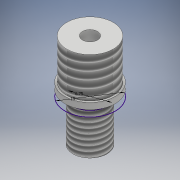
# Autodesk Inventor part: cuvette_holder_fiber_optics_connector
Saved by Autodesk Inventor 2017 (Build 210142000, 142)
## iProperties
Created: 2018-08-10
Part Number: cuvette_holder_fiber_optics_connector
Material: Generic
Document SubType Name: Modeling
Designer: qwertyuiop1
Density: 1 g/cm^3
Appearance: Default
Author: qwertyuiop1
Autodesk Inventor part; units mm, degrees
ref_plane "YZ Plane" through (0, 0, 0) normal (1, 0, 0) x (0, 1, 0)
ref_plane "XZ Plane" through (0, 0, 0) normal (0, 1, 0) x (-1, 0, 0)
ref_plane "XY Plane" through (0, 0, 0) normal (0, 0, 1) x (1, 0, 0)
sketch "Sketch1" plane through (0, 0, 0) normal (0, 0, 1) x (1, 0, 0)
  circle A0 centre (0, 0) radius 5
  dimension "d0" = 10
  constraints: 1 centre point, 1 coincident
  measures "d0" diameter of A0
extrude "Extrusion1" add sketch "Sketch1" along normal blind 18.75
sketch "Sketch2" plane through (0, 0, 18.75) normal (0, 0, 1) x (1, 0, 0)
  circle A0 centre (0, 0) radius 5
  circle A1 centre (0, 0) radius 4.625
  dimension "d3" = 9.25
  constraints: 2 centre point, 2 coincident
  measures "d3" diameter of A1
extrude "Extrusion2" cut sketch "Sketch2" against normal blind 8
sketch "Sketch3" plane through (0, 0, 18.75) normal (0, 0, 1) x (1, 0, 0)
  circle A0 centre (0, 0) radius 1.5
  dimension "d6" = 3
  constraints: 1 centre point, 1 coincident
  measures "d6" diameter of A0
extrude "Extrusion3" cut sketch "Sketch3" against normal blind 50
sketch "Sketch4" plane through (0, 0, 0) normal (0, 0, -1) x (-1, 0, 0)
  circle A0 centre (0, 0) radius 3.375
  circle A1 centre (0, 0) radius 5
  dimension "d9" = 6.75
  dimension "d10" = 10
  constraints: 2 centre point, 2 coincident
  measures "d9" diameter of A0
  measures "d10" diameter of A1
extrude "Extrusion4" cut sketch "Sketch4" against normal blind 8.25
sketch "Sketch5" plane through (0, 0, 8.25) normal (0, 0, -1) x (-1, 0, 0)
  circle A0 centre (0, 0) radius 3.375
  circle A1 centre (0, 0) radius 3.375 projected
  circle A2 centre (0, 0) radius 5
  dimension "d13" = 6.75
  dimension "d14" = 10
  constraints: 2 centre point, 2 coincident
  measures "d13" diameter of A0
  measures "d14" diameter of A2
thread "Thread1" size "M7x1" class "6g" standard "ANSI Metric M Profile" full length
thread "Thread2" size "M10x1.5" class "6g" standard "ANSI Metric M Profile" full length
sketch "Sketch6" plane through (0, 0, 8.25) normal (0, 0, -1) x (-1, 0, 0)
  circle A0 centre (0, 0) radius 3.375
  circle A1 centre (0, 0) radius 5
  constraints: 2 centre point, 2 coincident
extrude "Extrusion5" cut sketch "Sketch6" against normal blind 1.25
body "Solid1"
